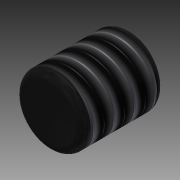
# Autodesk Inventor part: SetScrew
Saved by Autodesk Inventor 2014 SP1 (Build 180222100, 222)
## iProperties
Created: 2015-04-11
Part Number: SetScrew
Material: Aluminum 6061
Document SubType Name: Modeling
Designer: david
Mass: 0.0403157 g
Surface Area: 0.400011 cm^2
Volume: 0.0148766 cm^3
Density: 2.71 g/cm^3
Appearance: Aluminum - Polished
Author: david
Autodesk Inventor part; units mm, degrees
ref_plane "YZ Plane" through (0, 0, 0) normal (1, 0, 0) x (0, 1, 0)
ref_plane "XZ Plane" through (0, 0, 0) normal (0, 1, 0) x (-1, 0, 0)
ref_plane "XY Plane" through (0, 0, 0) normal (0, 0, 1) x (1, 0, 0)
sketch "Sketch1" plane through (0, 0, 0) normal (0, 1, 0) x (-1, 0, 0)
  circle A0 centre (0, 0) radius 1.321
  dimension "d2" = 2.642
  constraints: 1 centre point, 1 coincident
  measures "d2" diameter of A0
extrude "Extrusion1" add sketch "Sketch1" along normal blind 3.175
thread "Thread1" size "6-32 UNC" class "2A" standard "ANSI Unified Screw Threads" full length
sketch "Sketch2" plane through (0, 3.175, 0) normal (0, 1, 0) x (1, 0, 0)
  circle A0 centre (0, 0) radius 1.321 projected
  line L0 (0.9165, 0) -> (0.4583, -0.7937)
  line L1 (0.4583, -0.7937) -> (-0.4583, -0.7937)
  line L2 (-0.4583, -0.7937) -> (-0.9165, 0)
  line L3 (-0.9165, 0) -> (-0.4583, 0.7937)
  line L4 (-0.4583, 0.7937) -> (0.4583, 0.7937)
  line L5 (0.4583, 0.7937) -> (0.9165, 0)
  dimension "d9" = 1.5875
  constraints: 12 end point, 1 coincident, 13 other
  measures "d9" distance between parallel lines of L0 L3
fillet "Fillet1" radius 0.3 2 edges at (1.321, 3.175, 0) (1.321, 0, 0)
extrude "Extrusion2" cut sketch "Sketch2" against normal blind 1 contours L0 L1 L2 L3 L4 L5
fillet "Fillet2" radius 0.2 6 edges at (0.9165, 2.675, 0) (0.4583, 2.675, 0.7937) (0.4583, 2.675, -0.7937) (-0.4583, 2.675, -0.7937) (-0.9165, 2.675, 0) (-0.4583, 2.675, 0.7937)
fillet "Fillet3" radius 0.2 12 edges at (0.8856, 3.175, 0) (0.6874, 3.175, 0.3969) (0.4428, 3.175, 0.767) (0, 3.175, 0.7937) (-0.4428, 3.175, 0.767) (-0.6874, 3.175, 0.3969) (-0.8856, 3.175, 0) (-0.6874, 3.175, -0.3969) (-0.4428, 3.175, -0.767) (0, 3.175, -0.7937) (0.4428, 3.175, -0.767) (0.6874, 3.175, -0.3969)
body "Solid1"
